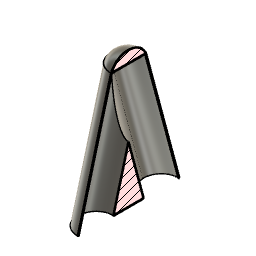
Knee (Autodesk Fusion 360 design; units mm, degrees)
Autodesk Fusion 360 part; units mm, degrees
sketch "Sketch1" plane through (0, 0, 0) normal (1, 0, 0) x (0, 1, 0)
  line L0 (0, 193.1852) -> (-51.7638, 0)
  line L1 (0, 193.1852) -> (51.7638, 0)
  line L2 (-150, 0) -> (150, 0) construction
  line L3 (0, 0) -> (0, 250) construction
  dimension "d1" = 200
  dimension "d3" = 200
  dimension "d4" = 30
  dimension "d5" = 250
  constraint horizontal L2
  constraint coincident L1.end L2
  constraint coincident L0.end L2
  constraint coincident L3.start origin
  constraint perpendicular L2 L3
  constraint coincident L0.start L3
  measures "d1" distance of L0.start L0.end
  measures "d3" distance of L0.start L1.end
  measures "d4" angle of L0 L1
  measures "d5" distance of L3.start L3.end
pipe "Pipe1" add diameter 53.04 wall 1.12 path "Sketch1" along L0 L1
ref_plane "WorkPlane1" through (0, 0, 10) normal (0, 0, 1) x (1, 0, 0)
sketch "Sketch2" plane through (0, 0, 10) normal (0, 0, 1) x (1, 0, 0)
  line L0 (250, 250) -> (-250, 250)
  line L1 (-250, 250) -> (-250, -250)
  line L2 (-250, -250) -> (250, -250)
  line L3 (250, -250) -> (250, 250)
  line L4 (250, 250) -> (-250, -250) construction
  line L5 (-250, 250) -> (250, -250) construction
  dimension "d11" = 500
  dimension "d12" = 500
  constraint horizontal L0
  constraint perpendicular L0 L1
  constraint parallel L0 L2
  constraint parallel L1 L3
  constraint coincident L4 origin
  constraint coincident L5 origin
  measures "d11" distance of L1.end L2.end
  measures "d12" distance of L0.end L1.end
extrude "Extrude1" cut sketch "Sketch2" against normal blind 500
ref_plane "WorkPlane2" through (0, 0, 197.5) normal (0, 0, 1) x (1, 0, 0)
sketch "Sketch3" plane through (0, 0, 197.5) normal (0, 0, 1) x (1, 0, 0)
  circle A0 centre (0, 0) radius 150
  dimension "d16" = 300
  constraint coincident A0.centre origin
  measures "d16" diameter of A0
extrude "Extrude2" cut sketch "Sketch3" along normal blind 150
sketch "Sketch5" plane through (0, 0, 197.5) normal (0, 0, 1) x (1, 0, 0)
  ellipse E0 centre (0, 1.1562) end of major axis (0, -25.1399) minor radius 25.4 (-25.3754, 0) -> (25.3754, 0) ccw
  ellipse E1 centre (0, 1.1562) end of major axis (0, -26.2994) minor radius 26.52 (-26.4965, 0) -> (26.4965, 0) ccw
  line L0 (-26.4965, 0) -> (-25.3754, 0)
  line L1 (25.3754, 0) -> (26.4965, 0)
ref_plane "WorkPlane3" through (26.52, 0, 0) normal (1, 0, 0) x (0, 1, 0)
sketch "Sketch6" plane through (26.52, 0, 0) normal (1, 0, 0) x (0, 1, 0)
  line L0 (0, 193.1852) -> (-51.7638, 0)
  line L1 (0, 193.1852) -> (51.7638, 0)
  line L2 (76.5398, 10) -> (21.6288, 10)
  line L3 (-21.6288, 10) -> (-76.5398, 10)
  line L4 (-21.6288, 10) -> (21.6288, 10)
  constraint coincident L3.start L4.start
  constraint coincident L2.end L4.end
extrude "Extrude3" add sketch "Sketch6" against normal blind 53
pipe "Pipe2" cut diameter 50.8 path "Sketch1" along L1 L0
sketch "Sketch7" plane through (0, 0, 0) normal (1, 0, 0) x (0, 1, 0)
  line L0 (0, 197.5) -> (-25.1399, 197.5)
  line L1 (25.1399, 197.5) -> (0, 197.5)
  line L2 (0, 187.5595) -> (-47.5769, 10)
  line L3 (-47.5769, 10) -> (-76.5398, 10)
  line L4 (-49.0843, 10) -> (0, 193.1852)
  line L5 (-26.2994, 197.5) -> (0, 197.5)
  line L6 (0, 197.5) -> (0, 193.1852)
  line L7 (47.5769, 10) -> (0, 187.5595)
  line L8 (0, 193.1852) -> (0, 187.5595)
  line L9 (0, 197.5) -> (26.2994, 197.5)
  line L10 (0, 193.1852) -> (49.0843, 10)
  line L11 (76.5398, 10) -> (47.5769, 10)
  line L12 (0, 197.5) -> (0, 215)
  arc A0 (0, 215) -> (-26.2994, 197.5) centre (-0.306, 186.9482) ccw
  line L13 (0, 193.1852) -> (0, 187.5595)
  line L14 (0, 197.5) -> (0, 193.1852)
  line L15 (0, 197.5) -> (0, 193.1852)
  line L16 (0, 197.5) -> (0, 193.1852)
  point P0 (0, 197.5)
  dimension "d29" = 17.5
  constraint coincident P0 L0.start
  constraint perpendicular L9 L12
  constraint coincident L5.start A0.end
  measures "d29" distance of P0 L12.end
revolve "Revolve4" add sketch "Sketch7" angle 360 about axis through (0, 0, 197.5) along (0, 0, 1) contours L0 L5 L12 A0
equation "d8 = 2 in + 2.24 mm"
